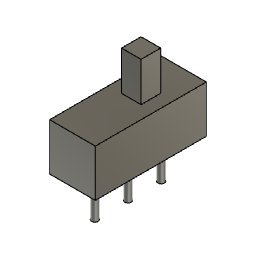
slide_SPDT (Autodesk Fusion 360 design; units mm, degrees)
Autodesk Fusion 360 part; units mm, degrees
sketch "スケッチ1" plane through (0, 0, 0) normal (0, 0, 1) x (1, 0, 0)
  line L0 (-1.75, -4.25) -> (1.75, -4.25)
  line L1 (1.75, -4.25) -> (1.75, 4.25)
  line L2 (1.75, 4.25) -> (-1.75, 4.25)
  line L3 (-1.75, 4.25) -> (-1.75, -4.25)
  line L4 (0, 1.75) -> (0, 22.5)
  line L5 (1.75, 0) -> (22.5, 0)
  circle A0 centre (0, 0) radius 0.25
  dimension "d1" = 3.5
  dimension "d2" = 8.5
  dimension "d9" = 0.5
  constraint horizontal L0
  constraint vertical L1
  constraint horizontal L2
  constraint vertical L3
  constraint symmetric L0 L2 L5
  constraint symmetric L1 L3 L4
  constraint coincident A0.centre origin
  measures "d1" distance of L0.start L0.end
  measures "d2" distance of L0.start L2.end
  measures "d9" diameter of A0
extrude "押し出し1" add sketch "スケッチ1" along normal blind 3.6 contours L0 L1 L2 L3 | A0
sketch "スケッチ2" plane through (0, 0, 3.6) normal (0, 0, 1) x (-1, 0, 0)
  line L0 (1.75, -4.25) -> (1.75, 4.25)
  line L1 (1.75, 4.25) -> (-1.75, 4.25)
  line L2 (-1.75, 4.25) -> (-1.75, -4.25)
  line L3 (-1.75, -4.25) -> (1.75, -4.25)
  line L4 (0.75, -1.75) -> (-0.75, -1.75)
  line L5 (-0.75, -1.75) -> (-0.75, -0.25)
  line L6 (-0.75, -0.25) -> (0.75, -0.25)
  line L7 (0.75, -0.25) -> (0.75, -1.75)
  line L8 (-1.75, 0) -> (-22.5, 0)
  line L9 (0, -1.75) -> (0, -22.5)
  dimension "d5" = 1.5
  dimension "d6" = 1.5
  dimension "d16" = 1.75
  constraint horizontal L4
  constraint vertical L5
  constraint horizontal L6
  constraint vertical L7
  constraint symmetric L5 L7 L9
  measures "d5" distance of L4.start L4.end
  measures "d6" distance of L4.start L6.end
  measures "d16" distance of origin L4
extrude "押し出し2" add sketch "スケッチ2" along normal blind 3 contours L4 L5 L6 L7
extrude "押し出し3" add sketch "スケッチ1" against normal blind 3 contours A0
pattern_linear "R パターン1" count 3 spacing 2.54 along (0, -1, 0) both ways of "押し出し3"
